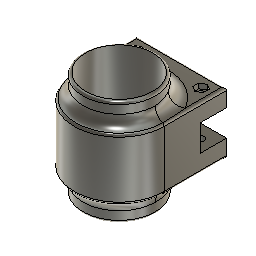
SuporteMotor (Autodesk Fusion 360 design; units mm, degrees)
Autodesk Fusion 360 part; units mm, degrees
sketch "Esboço1" plane through (0, 0, 0) normal (0, 0, 1) x (1, 0, 0)
  circle A0 centre (0, 0) radius 19
  circle A1 centre (0, 0) radius 20.5
  dimension "d1" = 38
  dimension "d2" = 41
  constraint coincident A0.centre A1.centre
  constraint concentric A0 A1
  measures "d1" diameter of A0
  measures "d2" diameter of A1
extrude "Extrusão1" add sketch "Esboço1" along normal blind 60
extrude "Extrusão2" add sketch "Esboço1" along normal blind 3 contours A0
sketch "Esboço2" plane through (0, 0, 0) normal (0, 0, 1) x (1, 0, 0)
  circle A0 centre (15, 0) radius 2
  circle A1 centre (7.5, 12.9904) radius 2
  circle A2 centre (-7.5, 12.9904) radius 2
  circle A3 centre (-15, 0) radius 2
  circle A4 centre (-7.5, -12.9904) radius 2
  circle A5 centre (7.5, -12.9904) radius 2
  dimension "d7" = 15
  dimension "d8" = 4
  dimension "d10" = 360
  measures "d7" distance of origin A0.centre
  measures "d8" diameter of A0
extrude "Extrusão3" cut sketch "Esboço2" along normal blind 11
sketch "Esboço3" plane through (0, 0, 0) normal (0, 0, 1) x (1, 0, 0)
  circle A0 centre (0, 7) radius 6.5
  dimension "d13" = 7
  dimension "d14" = 13
  measures "d13" distance of origin A0.centre
  measures "d14" diameter of A0
extrude "Extrusão4" cut sketch "Esboço3" along normal blind 24
sketch "Esboço4" plane through (0, 0, 0) normal (0, 0, 1) x (1, 0, 0)
  line L0 (-20.5, 0) -> (-25.5, 0)
  line L1 (-25.5, 0) -> (-25.5, 35.5)
  circle A0 centre (0, 0) radius 20.5
  line L2 (-20.5, 35.5) -> (-25.5, 35.5)
  line L3 (20.5, 0) -> (25.5, 0)
  line L4 (25.5, 0) -> (25.5, 35.5)
  line L5 (25.5, 35.5) -> (20.5, 35.5)
  line L6 (20.5, 35.5) -> (-20.5, 35.5)
  arc A1 (-25.5, 0) -> (25.5, 0) centre (0, 0) ccw
  dimension "d17" = 5
  dimension "d19" = 5
  constraint horizontal L0
  constraint vertical L1
  constraint coincident L0.start A0
  constraint perpendicular L1 L2
  constraint coincident A0 L3.start
  constraint parallel L0 L3
  constraint perpendicular L2 L4
  constraint perpendicular L4 L5
  constraint coincident L2.start L6.end
  constraint coincident L5.end L6.start
  measures "d17" distance of L0.start L0.end
  measures "d19" distance of L3.start L3.end
extrude "Extrusão9" add sketch "Esboço4" along normal mid plane 35 from surface at 30 contours L0 A0 L3 A1 | L0 L1 A0 L2 L3 L4 L5 L6
sketch "Esboço5" plane through (25.5, 0, 0) normal (1, 0, 0) x (0, 1, 0)
  line L0 (35.5, 12.5) -> (35.5, 47.5)
  line L1 (35.5, 47.5) -> (0, 47.5)
  line L2 (0, 47.5) -> (0, 12.5)
  line L3 (0, 12.5) -> (35.5, 12.5)
  line L4 (35.5, 37.5) -> (20.5, 37.5)
  line L5 (20.5, 37.5) -> (20.5, 22.5)
  line L6 (20.5, 22.5) -> (35.5, 22.5)
  line L7 (35.5, 37.5) -> (35.5, 22.5)
  dimension "d35" = 15
  constraint perpendicular L4 L5
  constraint perpendicular L0 L6
  constraint perpendicular L6 L7
  measures "d35" distance of L4.start L4.end
extrude "Extrusão10" cut sketch "Esboço5" against normal blind 59 contours L0 L4 L5 L6 L7
sketch "Esboço6" plane through (0, 0, 47.5) normal (0, 0, 1) x (-1, 0, 0)
  circle A0 centre (0, 0) radius 20.5
  arc A1 (25.5, 0) -> (-25.5, 0) centre (0, 0) ccw
  line L0 (-25.5, 0) -> (-25.5, -35.5)
  line L1 (-25.5, -35.5) -> (25.5, -35.5)
  line L2 (25.5, -35.5) -> (25.5, 0)
  circle A2 centre (-18.5, -28) radius 2
  circle A3 centre (18.5, -28) radius 2
  dimension "d42" = 4
  dimension "d43" = 4
  measures "d42" diameter of A2
  measures "d43" diameter of A3
extrude "Extrusão11" cut sketch "Esboço6" against normal blind 43 contours A2 | A3
sketch "Esboço7" plane through (0, 0, 47.5) normal (0, 0, 1) x (-1, 0, 0)
  circle A0 centre (-18.5, -28) radius 2
  circle A1 centre (18.5, -28) radius 2
  circle A2 centre (0, 0) radius 20.5
  arc A3 (25.5, 0) -> (-25.5, 0) centre (0, 0) ccw
  line L0 (-25.5, 0) -> (-25.5, -35.5)
  line L1 (-25.5, -35.5) -> (25.5, -35.5)
  line L2 (25.5, -35.5) -> (25.5, 0)
  line L3 (-15.5, -26.2679) -> (-18.5, -24.5359)
  line L4 (-18.5, -24.5359) -> (-21.5, -26.2679)
  line L5 (-21.5, -26.2679) -> (-21.5, -29.7321)
  line L6 (-21.5, -29.7321) -> (-18.5, -31.4641)
  line L7 (-18.5, -31.4641) -> (-15.5, -29.7321)
  line L8 (-15.5, -29.7321) -> (-15.5, -26.2679)
  line L9 (21.4679, -29.7865) -> (21.5311, -26.3229)
  line L10 (21.5311, -26.3229) -> (18.5632, -24.5365)
  line L11 (18.5632, -24.5365) -> (15.5321, -26.2135)
  line L12 (15.5321, -26.2135) -> (15.4689, -29.6771)
  line L13 (15.4689, -29.6771) -> (18.4368, -31.4635)
  line L14 (18.4368, -31.4635) -> (21.4679, -29.7865)
  point P0 (-18.5, -28)
  point P1 (18.5, -28)
  dimension "d46" = 3
  dimension "d47" = 3
  constraint coincident P0 A0.centre
  constraint coincident P1 A1.centre
  measures "d46" distance of P0 L8
  measures "d47" distance of P1 L14
extrude "Extrusão12" cut sketch "Esboço7" against normal blind 2.8 contours L3 L4 L5 L6 L7 L8 | L9 L10 L11 L12 L13 L14
chamfer "Chanfro1" distance 1.5 distance2 1.5 2 edges at (20.3647, 28.7232, 12.5) (-16.6353, 28.7232, 12.5) measured on face at (0.5107, 26.232, 12.5) measured on face at (0.5107, 26.232, 12.5)
fillet "Arredondamento1" radius 1.5 10 edges at (-25.5, 17.75, 47.5) (0, -25.5, 47.5) (25.5, 17.75, 47.5) (25.5, 17.75, 12.5) (0, -25.5, 12.5) (-25.5, 17.75, 12.5) (0, 35.5, 47.5) (0, 35.5, 12.5) (-19.1127, -7.4131, 60) (-19.1127, -7.4131, 0)
fillet "Arredondamento2" radius 7 2 edges at (-19.1127, -7.4131, 47.5) (-19.1127, 7.4131, 12.5)
equation "d17 = d19"
equation "d46 = ( ( 5 / 2 ) * 1 mm ) + 0.5 * 1 mm"
equation "d47 = d46"
